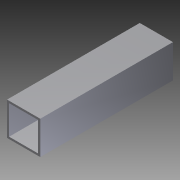
# Autodesk Inventor part: 1-16 tube 4''
Saved by Autodesk Inventor 2011 SP1 (Build 150282100, 282)
## iProperties
Created: 2013-01-18
Part Number: 1-16 tube 4''
Document SubType Name: Modeling
Designer: wes
Density: 1 g/cm^3
Author: wes
Autodesk Inventor part; units mm, degrees
ref_plane "YZ Plane" through (0, 0, 0) normal (1, 0, 0) x (0, 1, 0)
ref_plane "XZ Plane" through (0, 0, 0) normal (0, 1, 0) x (-1, 0, 0)
ref_plane "XY Plane" through (0, 0, 0) normal (0, 0, 1) x (1, 0, 0)
sketch "Sketch1" plane through (0, 0, 0) normal (0, 0, 1) x (1, 0, 0)
  line L0 (-18.9528, 7.3952) -> (6.4472, 7.3952)
  line L1 (6.4472, 7.3952) -> (6.4472, -18.0048)
  line L2 (6.4472, -18.0048) -> (-18.9528, -18.0048)
  line L3 (-18.9528, -18.0048) -> (-18.9528, 7.3952)
  line L4 (-17.3653, 5.8077) -> (4.8597, 5.8077)
  line L5 (4.8597, 5.8077) -> (4.8597, -16.4173)
  line L6 (4.8597, -16.4173) -> (-17.3653, -16.4173)
  line L7 (-17.3653, -16.4173) -> (-17.3653, 5.8077)
  point P0 (0, 0)
  dimension "d0" = 25.4
  dimension "d1" = 25.4
  dimension "d2" = 1.5875
  dimension "d3" = 1.5875
  dimension "d4" = 1.5875
  dimension "d5" = 1.5875
  constraints: 16 end point, 4 parallel, 2 horizontal, 2 perpendicular
  measures "d0" distance of L0.start L0.end
  measures "d1" distance of L2.end L0.start
  measures "d2" distance between parallel lines of L7 L3
  measures "d3" distance between parallel lines of L1 L5
  measures "d4" distance between parallel lines of L0 L4
  measures "d5" distance between parallel lines of L2 L6
extrude "Extrusion1" add sketch "Sketch1" along normal blind 101.6
body "Solid1"
